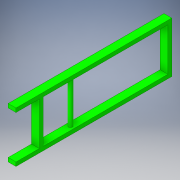
# Autodesk Inventor part: stage
Saved by Autodesk Inventor 2016 (Build 200138000, 138)
## iProperties
Created: 2018-01-19
Part Number: stage
Material: Generic
Document SubType Name: Modeling
Designer: New User
Density: 1 g/cm^3
Appearance: Default
Author: New User
Autodesk Inventor part; units mm, degrees
note: some values were not read from the file. Chosen so that the rebuilt part matches the saved one: second side of "Extrusion4".
ref_plane "YZ Plane" through (0, 0, 0) normal (1, 0, 0) x (0, 1, 0)
ref_plane "XZ Plane" through (0, 0, 0) normal (0, 1, 0) x (-1, 0, 0)
ref_plane "XY Plane" through (0, 0, 0) normal (0, 0, 1) x (1, 0, 0)
sketch "Sketch1" plane through (0, 0, 0) normal (0, 1, 0) x (-1, 0, 0)
  line L0 (0, 0) -> (-50.8, 0)
  line L1 (-50.8, 0) -> (-50.8, 1016)
  line L2 (-50.8, 1016) -> (0, 1016)
  line L3 (0, 1016) -> (0, 0)
  dimension "d0" = 1016
  dimension "d1" = 50.8
  constraints: 8 end point, 2 parallel, 1 horizontal, 1 perpendicular
  measures "d0" distance of L2.end L0.start
  measures "d1" distance of L1.end L2.end
extrude "Extrusion1" add sketch "Sketch1" along normal blind 25.4
sketch "Sketch2" plane through (0, 0, 0) normal (0, -1, 0) x (1, 0, 0)
  line L0 (0, 838.2) -> (50.8, 838.2)
  line L1 (50.8, 838.2) -> (50.8, 863.6)
  line L2 (50.8, 863.6) -> (0, 863.6)
  line L3 (0, 863.6) -> (0, 838.2)
  line L4 (50.8, 1016) -> (0, 1016) projected
  line L5 (50.8, 0) -> (0, 0) projected
  line L6 (50.8, 0) -> (0, 0)
  line L7 (0, 0) -> (0, 25.4)
  line L8 (0, 25.4) -> (50.8, 25.4)
  line L9 (50.8, 25.4) -> (50.8, 0)
  dimension "d4" = 25.4
  dimension "d7" = 152.4
  dimension "d30" = 25.4
  constraints: 16 end point, 4 parallel, 2 horizontal, 2 perpendicular
  measures "d4" distance of L2.end L0.start
  measures "d7" distance between parallel lines of L2 L4
  measures "d30" distance of L8.end L5.start
extrude "Extrusion2" add sketch "Sketch2" along normal blind 279.4
sketch "Sketch3" plane through (0, -279.4, 0) normal (0, -1, 0) x (1, 0, 0)
  line L0 (50.8, 0) -> (0, 0) projected
  line L1 (0, 1016) -> (50.8, 1016) projected
  line L2 (0, 0) -> (50.8, 0)
  line L3 (50.8, 0) -> (50.8, 1016)
  line L4 (50.8, 1016) -> (0, 1016)
  line L5 (0, 1016) -> (0, 0)
  constraints: 8 end point, 2 parallel, 1 horizontal, 1 perpendicular
extrude "Extrusion3" add sketch "Sketch3" along normal blind 25.4
sketch "Sketch4" plane through (0, -279.4, 0) normal (0, 1, 0) x (1, 0, 0)
  circle A0 centre (25.4, -635) radius 12.7
  line L0 (0, -1016) -> (50.8, -1016) projected
  line L1 (0, -1016) -> (0, -863.6) projected
  point P0 (0, 0)
  dimension "d12" = 25.4
  dimension "d13" = 381
  dimension "d18" = 25.4
  constraints: 1 centre point
  measures "d12" diameter of A0
  measures "d13" distance from line of L0 A0.centre
  measures "d18" distance from line of L1 A0.centre
extrude "Extrusion4" add sketch "Sketch4" along normal blind 284.1625
body "Solid1"
